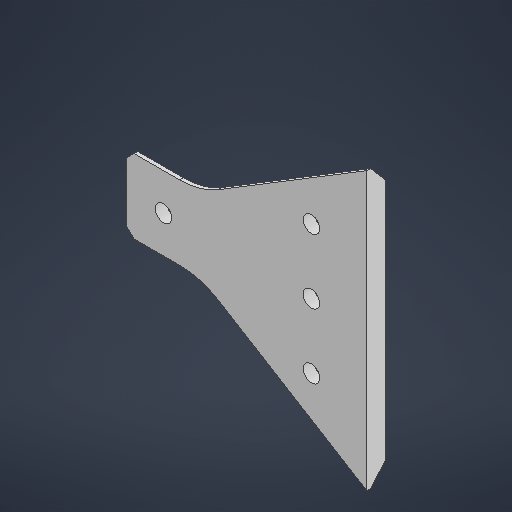
# Autodesk Inventor part: Y Axis Holder
Saved by Autodesk Inventor 2025.1 (Build 291241000, 241)
## iProperties
Created: 2025-02-22
Part Number: Y Axis Holder
Material: Generic
Document SubType Name: Modeling
Designer: jerem
Density: 1 g/cm^3
Appearance: Default
Author: jerem
## iProperties of the stored document Y Axis Holder_3DPrint.ipt
Created: 2025-02-22
Part Number: Y Axis Holder_3DPrint
Material: Generic
Document SubType Name: Modeling
Designer: jerem
Density: 1 g/cm^3
Appearance: Default
Author: jerem
Autodesk Inventor part; units mm, degrees
ref_plane "YZ Plane" through (0, 0, 0) normal (1, 0, 0) x (0, 1, 0)
ref_plane "XZ Plane" through (0, 0, 0) normal (0, 1, 0) x (-1, 0, 0)
ref_plane "XY Plane" through (0, 0, 0) normal (0, 0, 1) x (1, 0, 0)
sketch "Sketch1" plane through (0, 0, 0) normal (0, 0, 1) x (1, 0, 0)
  line L0 (0, 0) -> (-50, 0) construction
  line L1 (-50, 0) -> (-50, 10)
  line L2 (-50, 0) -> (-50, -10)
  line L3 (-50, -10) -> (-30, -10)
  line L4 (-30, -10) -> (15, -37.5)
  line L5 (-50, 10) -> (-30, 10)
  line L6 (-30, 10) -> (15, 37.5)
  line L7 (15, 37.5) -> (15, -37.5)
  line L8 (0, 0) -> (15, 0) construction
  line L9 (0, 17.5) -> (0, -17.5) construction
  point P0 (-40, 0)
  dimension "d0" = 20
  dimension "d1" = 65
  dimension "d2" = 50
  dimension "d4" = 20
  dimension "d5" = 75
  dimension "d6" = 35
  dimension "d9" = 40
  constraints: 20 end point, 3 coincident, 3 equal length, 3 vertical, 2 horizontal, 2 midpoint, 2 perpendicular, 1 point on line
  measures "d0" distance between parallel lines of L3 L5
  measures "d1" distance of L8.end L0.end
  measures "d2" distance between parallel lines of L1 L9
  measures "d4" distance of L1.end L5.end
  measures "d5" distance of L6.end L4.end
  measures "d6" distance of L9.end L9.start
  measures "d9" distance of L0.start point (-40, 0)
extrude "Extrusion1" add sketch "Sketch1" along normal blind 5
hole "Hole1" at (0, 17.5, 0) at (0, -17.5, 0) at (-40, 0, 0) at (0, 0, 0) direction (0, 0, 1) diameter 4.5 end through all counterbore diameter 8 counterbore depth 2
fillet "Fillet1" radius 20 2 edges at (-30, 10, 2.5) (-30, -10, 2.5)
chamfer "Chamfer1" distance 2 angle 45 2 edges at (-50, 10, 2.5) (-50, -10, 2.5)
chamfer "Chamfer2" distance 4 angle 45 6 edges at (-41.8137, 10, 0) (-30.2103, 10.7476, 0) (-5.0992, 25.2172, 0) (-30.2103, -10.7476, 0) (-5.0992, -25.2172, 0) (-41.8137, -10, 0)
body "Solid1"
